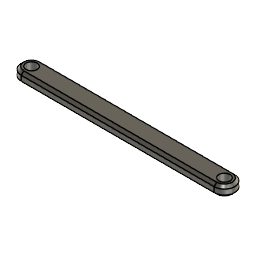
Softy.Gripper.1.0 (Autodesk Fusion 360 archive; units mm, degrees)
design "Support"
part number: 2026-04-04-04-06-12-103
Autodesk Fusion 360 part; units mm, degrees
sketch "Sketch1" plane through (0, 0, 0) normal (0, 0, 1) x (1, 0, 0)
  circle A0 centre (0, 0) radius 2.15
  circle A1 centre (0, 0) radius 4
  circle A2 centre (-74.481, 0) radius 2.15
  circle A3 centre (-74.481, 0) radius 4
  line L0 (0, 4) -> (-74.481, 4)
  line L1 (-74.481, -4) -> (0, -4)
  dimension "d1" = 4.3
  dimension "d2" = 8
  dimension "d3" = 74.481
  dimension "d4" = 4.3
  dimension "d5" = 8
  constraint coincident A0.centre A1.centre
  constraint concentric A0 A1
  constraint coincident A1 L0.start
  constraint concentric A2 A3
  constraint coincident A3 L0.end
  constraint tangent A3 L0
  constraint coincident A3 L1.start
  constraint coincident A1 L1.end
  constraint tangent A1 L1
  constraint horizontal L1
  measures "d1" diameter of A0
  measures "d2" diameter of A1
  measures "d3" distance of A0.centre A2.centre
  measures "d4" diameter of A2
  measures "d5" diameter of A3
extrude "Extrude1" add sketch "Sketch1" along normal blind 4
chamfer "Chamfer1" distance 1 angle 45 8 edges at (-37.2405, -4, 4) (4, 0, 4) (-37.2405, 4, 4) (-78.481, 0, 4) (-78.481, 0, 0) (-37.2405, -4, 0) (4, 0, 0) (-37.2405, 4, 0)

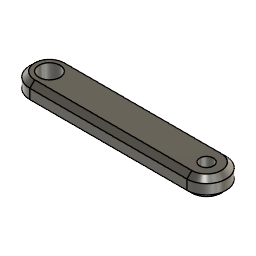
design "ServoSupport"
part number: 2026-04-04-15-48-57-134
Autodesk Fusion 360 part; units mm, degrees
sketch "Sketch1" plane through (0, 0, 0) normal (0, 0, 1) x (1, 0, 0)
  circle A0 centre (0, 0) radius 1.4
  circle A1 centre (0, 0) radius 4
  circle A2 centre (-32, 0) radius 2.15
  circle A3 centre (-32, 0) radius 4
  line L0 (-32, 4) -> (0, 4)
  line L1 (0, -4) -> (-32, -4)
  dimension "d1" = 2.8
  dimension "d2" = 8
  dimension "d3" = 32
  dimension "d4" = 4.3
  dimension "d5" = 8
  constraint coincident A0.centre A1.centre
  constraint concentric A2 A3
  constraint coincident A3 L0.start
  constraint coincident A1 L0.end
  constraint tangent A1 L0
  constraint coincident A1 L1.start
  constraint coincident A3 L1.end
  constraint tangent A3 L1
  measures "d1" diameter of A0
  measures "d2" diameter of A1
  measures "d3" distance of A0.centre A2.centre
  measures "d4" diameter of A2
  measures "d5" diameter of A3
extrude "Extrude1" add sketch "Sketch1" along normal blind 4
chamfer "Chamfer1" distance 1 angle 45 8 edges at (-16, -4, 4) (4, 0, 4) (-16, 4, 4) (-36, 0, 4) (-16, -4, 0) (-36, 0, 0) (-16, 4, 0) (4, 0, 0)

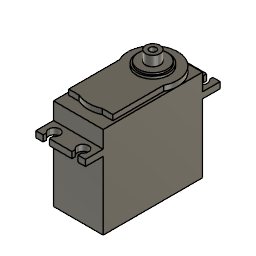
design "MG995"
part number: 2026-04-01-22-42-17-467
Autodesk Fusion 360 part; units mm, degrees
sketch "Sketch1" plane through (0, 0, 0) normal (0, 0, 1) x (1, 0, 0)
  line L0 (-10, 20) -> (10, 20)
  line L1 (10, 20) -> (10, -20)
  line L2 (10, -20) -> (-10, -20)
  line L3 (-10, -20) -> (-10, 20)
  line L4 (-10, 20) -> (10, -20) construction
  line L5 (10, 20) -> (-10, -20) construction
  dimension "d1" = 20
  dimension "d2" = 40
  constraint horizontal L0
  constraint perpendicular L0 L1
  constraint parallel L0 L2
  constraint parallel L1 L3
  constraint coincident L4 origin
  constraint coincident L5 origin
  measures "d1" distance of L1.end L2.end
  measures "d2" distance of L0.end L1.end
extrude "Extrude1" add sketch "Sketch1" along normal blind 36.85
sketch "Sketch2" plane through (0, 0, 36.85) normal (0, 0, 1) x (-1, 0, 0)
  line L0 (10, 20) -> (-10, 20)
  line L1 (-10, 20) -> (-10, -20)
  line L2 (-10, -20) -> (10, -20)
  line L3 (10, -20) -> (10, 20)
  line L4 (8.9, 0) -> (8.9, 15)
  line L5 (-8.9, 0) -> (-8.9, 15)
  circle A0 centre (0, -10) radius 10
  line L6 (8.9, 0) -> (8.9, -5.4404)
  line L7 (-8.9, 0) -> (-8.9, -5.4404)
  arc A1 (4.675, 15) -> (-4.675, 15) centre (0, 4.5722) ccw
  line L8 (4.675, 15) -> (8.9, 15)
  line L9 (-4.675, 15) -> (-8.9, 15)
  dimension "d5" = 8.9
  dimension "d6" = 8.9
  dimension "d11" = 10
  constraint tangent L1 A0
  constraint coincident A0 L6.end
  constraint parallel L4 L6
  constraint coincident A0 L7.end
  constraint parallel L5 L7
  constraint perpendicular L4 L8
  constraint perpendicular L5 L9
  measures "d5" distance of origin L5.start
  measures "d6" distance of origin L4.start
  measures "d11" distance of origin A0.centre
extrude "Extrude2" add sketch "Sketch2" along normal blind 2.15 contours A0 | L4 L5 A0 L6 L7 A1 L8 L9
sketch "Sketch3" plane through (0, 0, 39) normal (0, 0, 1) x (-1, 0, 0)
  arc A0 (4.675, 15) -> (-4.675, 15) centre (0, 4.5722) ccw
  line L0 (-4.675, 15) -> (-8.9, 15)
  line L1 (-8.9, 15) -> (-8.9, -5.4404)
  arc A1 (-8.9, -5.4404) -> (8.9, -5.4404) centre (0, -10) ccw
  line L2 (8.9, -5.4404) -> (8.9, 15)
  line L3 (8.9, 15) -> (4.675, 15)
  line L4 (0, -20) -> (0, -10)
  circle A2 centre (0, -10) radius 6.5
  dimension "d15" = 10
  dimension "d16" = 13
  constraint midpoint A1 L4.start
  constraint vertical L4
  measures "d15" distance of L4.start A1.centre
  measures "d16" diameter of A2
extrude "Extrude3" add sketch "Sketch3" along normal blind 1 contours A2
sketch "Sketch4" plane through (0, 0, 40) normal (0, 0, 1) x (-1, 0, 0)
  circle A0 centre (0, -10) radius 6.5
  circle A1 centre (0, -10) radius 5.825
  dimension "d19" = 11.65
  constraint concentric A0 A1
  measures "d19" diameter of A1
extrude "Extrude4" add sketch "Sketch4" along normal blind 0.75 contours A1
sketch "Sketch5" plane through (0, 0, 40.75) normal (0, 0, 1) x (-1, 0, 0)
  circle A0 centre (0, -10) radius 5.825
  circle A1 centre (0, -10) radius 2.925
  dimension "d22" = 5.85
  constraint concentric A0 A1
  measures "d22" diameter of A1
extrude "Extrude5" add sketch "Sketch5" along normal blind 4 contours A1
sketch "Sketch6" plane through (0, 0, 44.75) normal (0, 0, 1) x (-1, 0, 0)
  circle A0 centre (0, -10) radius 2.925
  circle A1 centre (0, -10) radius 1.35
  dimension "d25" = 2.7
  constraint concentric A0 A1
  measures "d25" diameter of A1
extrude "Extrude6" cut sketch "Sketch6" against normal blind 4 contours A1
sketch "Sketch7" plane through (0, -20, 0) normal (0, -1, 0) x (1, 0, 0)
  line L0 (-10, 0) -> (10, 0)
  line L1 (10, 0) -> (10, 36.85)
  line L2 (10, 36.85) -> (-10, 36.85)
  line L3 (-10, 36.85) -> (-10, 0)
  line L4 (-10, 30) -> (10, 30)
  line L5 (10, 30) -> (10, 27.5)
  line L6 (10, 27.5) -> (-10, 27.5)
  line L7 (-10, 27.5) -> (-10, 30)
  dimension "d29" = 2.5
  constraint horizontal L4
  constraint vertical L5
  constraint horizontal L6
  constraint vertical L7
  constraint coincident L3 L4.start
  measures "d29" distance of L4.start L6.end
extrude "Extrude7" add sketch "Sketch7" along normal blind 7.125 and the other way blind 47.125 contours L1 L3 L4 L5 L6 L7
sketch "Sketch8" plane through (0, 0, 30) normal (0, 0, 1) x (-1, 0, 0)
  line L0 (-10, 20) -> (10, 20)
  line L1 (10, 20) -> (10, 27.125)
  line L2 (10, 27.125) -> (-10, 27.125)
  line L3 (-10, 27.125) -> (-10, 20)
  circle A0 centre (5.775, 23.9) radius 2.225
  line L4 (0, -2.5) -> (0, -20)
  circle A1 centre (-5.775, 23.9) radius 2.225
  line L5 (5.775, 23.9) -> (5.775, 27.125)
  line L6 (5.775, 27.125) -> (7, 27.125)
  line L7 (5.775, 27.125) -> (4.55, 27.125)
  line L8 (-5.775, 23.9) -> (-5.775, 27.125)
  line L9 (-5.775, 27.125) -> (-4.55, 27.125)
  line L10 (-5.775, 27.125) -> (-7, 27.125)
  line L11 (-7, 27.125) -> (-7, 25.7574)
  line L12 (-4.55, 27.125) -> (-4.55, 25.7574)
  line L13 (4.55, 27.125) -> (4.55, 25.7574)
  line L14 (7, 27.125) -> (7, 25.7574)
  line L15 (-20, 0) -> (-2.5, 0)
  line L16 (5.775, -27.125) -> (7, -27.125)
  line L17 (5.775, -27.125) -> (4.55, -27.125)
  line L18 (4.55, -27.125) -> (4.55, -25.7574)
  line L19 (7, -27.125) -> (7, -25.7574)
  circle A2 centre (5.775, -23.9) radius 2.225
  circle A3 centre (-5.775, -23.9) radius 2.225
  line L20 (-7, -27.125) -> (-7, -25.7574)
  line L21 (-5.775, -27.125) -> (-4.55, -27.125)
  line L22 (-4.55, -27.125) -> (-4.55, -25.7574)
  line L23 (-5.775, -27.125) -> (-7, -27.125)
  dimension "d36" = 2.225
  dimension "d37" = 1.225
  dimension "d38" = 1.225
  dimension "d39" = 1.225
  dimension "d40" = 1.225
  constraint symmetric A0 L4 A1
  constraint coincident A0.centre L5.start
  constraint coincident L2 L5.end
  constraint perpendicular L2 L5
  constraint perpendicular L5 L6
  constraint perpendicular L5 L7
  constraint coincident A1.centre L8.start
  constraint coincident L2 L8.end
  constraint perpendicular L2 L8
  constraint perpendicular L8 L9
  constraint perpendicular L8 L10
  constraint coincident A1 L11.end
  constraint perpendicular L10 L11
  constraint coincident A1 L12.end
  constraint perpendicular L9 L12
  constraint coincident A0 L13.end
  constraint perpendicular L7 L13
  constraint coincident A0 L14.end
  constraint perpendicular L6 L14
  constraint symmetric A0 L15 A2
  constraint symmetric A1 L15 A3
  constraint symmetric L5.end L15 L16.start
  constraint symmetric L6.end L15 L16.end
  constraint symmetric L7.end L15 L17.end
  constraint symmetric L8.end L15 L21.start
  constraint symmetric L9.end L15 L21.end
  constraint symmetric L10.end L15 L20.start
  constraint symmetric L11.end L15 L20.end
  constraint symmetric L12.end L15 L22.end
  constraint symmetric L13.end L15 L18.end
  constraint symmetric L14.end L15 L19.end
  measures "d36" radius of A0
  measures "d37" distance of L5.end L6.end
  measures "d38" distance of L5.end L7.end
  measures "d39" distance of L8.end L9.end
  measures "d40" distance of L8.end L10.end
extrude "Extrude8" cut sketch "Sketch8" against normal blind 2.5 contours L2 A1 L8 L10 L11 | L2 A0 L5 L6 L14 | L2 A1 L8 L9 L12 | A1 | L2 A0 L5 L7 L13 | A0 | L16 L17 L18 L19 A2 | A2 | A3 | A3 L20 L21 L22 L23

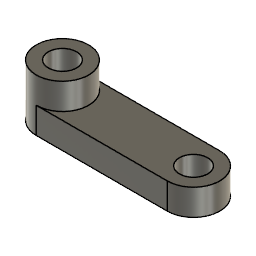
design "support_short"
part number: 2026-04-04-02-22-16-847
Autodesk Fusion 360 part; units mm, degrees
sketch "Sketch1" plane through (0, 0, 0) normal (0, 0, 1) x (1, 0, 0)
  circle A0 centre (0, 0) radius 2.15
  circle A1 centre (-20, 0) radius 2.15
  circle A2 centre (0, 0) radius 4
  circle A3 centre (-20, 0) radius 4
  line L0 (-20, 4) -> (0, 4)
  line L1 (0, -4) -> (-20, -4)
  dimension "d1" = 4.3
  dimension "d2" = 4.3
  dimension "d3" = 8
  dimension "d4" = 8
  constraint coincident A0.centre A2.centre
  constraint concentric A0 A2
  constraint concentric A1 A3
  constraint coincident A3 L0.start
  constraint coincident A2 L0.end
  constraint coincident A2 L1.start
  constraint coincident A3 L1.end
  measures "d1" diameter of A0
  measures "d2" diameter of A1
  measures "d3" diameter of A2
  measures "d4" diameter of A3
extrude "Extrude1" add sketch "Sketch1" along normal blind 4
extrude "Extrude2" add sketch "Sketch1" along normal blind 8 contours A3

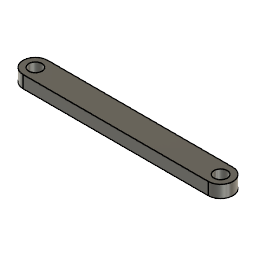
design "support_long"
part number: 2026-04-04-01-35-22-601
Autodesk Fusion 360 part; units mm, degrees
sketch "Sketch1" plane through (0, 0, 0) normal (0, 0, 1) x (1, 0, 0)
  circle A0 centre (0, 0) radius 2.15
  circle A1 centre (-60, 0) radius 2.15
  circle A2 centre (-60, 0) radius 4
  circle A3 centre (0, 0) radius 4
  line L0 (-60, 4) -> (0, 4)
  line L1 (0, -4) -> (-60, -4)
  dimension "d1" = 60
  dimension "d2" = 4.3
  dimension "d3" = 4.3
  dimension "d4" = 8
  dimension "d5" = 8
  constraint coincident A0.centre A3.centre
  constraint concentric A1 A2
  constraint concentric A0 A3
  constraint coincident A3 L0.end
  constraint coincident A3 L1.start
  constraint coincident A2 L0.start
  constraint coincident A2 L1.end
  measures "d1" distance of A0.centre A1.centre
  measures "d2" diameter of A0
  measures "d3" diameter of A1
  measures "d4" diameter of A2
  measures "d5" diameter of A3
extrude "Extrude1" add sketch "Sketch1" along normal blind 4
